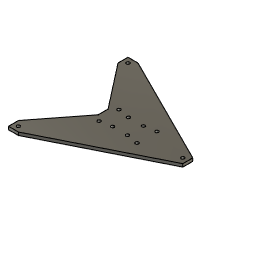
V0.1 Y Carriage (Autodesk Fusion 360 design; units mm, degrees)
Autodesk Fusion 360 part; units mm, degrees
sketch "Sketch1" plane through (0, 0, 0) normal (0, 0, 1) x (1, 0, 0)
  line L0 (60, -60) -> (-60, -60)
  line L1 (-60, -60) -> (-60, 60)
  line L2 (-60, 60) -> (60, 60)
  line L3 (60, 60) -> (60, -60)
  line L4 (60, -60) -> (-60, 60) construction
  line L5 (-60, -60) -> (60, 60) construction
  line L6 (25, 20) -> (-25, 20)
  line L7 (-25, 20) -> (-25, -20)
  line L8 (-25, -20) -> (25, -20)
  line L9 (25, -20) -> (25, 20)
  line L10 (25, 20) -> (-25, -20) construction
  line L11 (-25, 20) -> (25, -20) construction
  line L12 (60, 5) -> (-50, 60)
  line L13 (60, -5) -> (-50, -60)
  line L14 (-60, 50) -> (-25, 5)
  line L15 (-60, -50) -> (-25, -5)
  dimension "d1" = 120
  dimension "d2" = 120
  dimension "d6" = 50
  dimension "d7" = 40
  dimension "d29" = 5
  dimension "d30" = 5
  dimension "d31" = 10
  dimension "d34" = 10
  dimension "d41" = 10
  dimension "d42" = 10
  constraint horizontal L0
  constraint perpendicular L0 L1
  constraint parallel L0 L2
  constraint parallel L1 L3
  constraint coincident L4 origin
  constraint coincident L5 origin
  constraint horizontal L6
  constraint perpendicular L6 L7
  constraint parallel L6 L8
  constraint parallel L7 L9
  constraint coincident L10 origin
  constraint coincident L11 origin
  constraint coincident L3 L12.start
  constraint coincident L2 L12.end
  constraint coincident L3 L13.start
  constraint coincident L0 L13.end
  constraint coincident L1 L14.start
  constraint coincident L7 L14.end
  constraint coincident L1 L15.start
  constraint coincident L7 L15.end
  constraint horizontal L13.start L15.end
  constraint horizontal L12.start L14.end
  measures "d1" distance of L1.end L2.end
  measures "d2" distance of L0.end L1.end
  measures "d6" distance of L7.end L8.end
  measures "d7" distance of L6.end L7.end
  measures "d29" vertical distance of origin L12.start
  measures "d30" vertical distance of origin L13.start
  measures "d31" distance of L1.end L12.end
  measures "d34" distance of L0.end L13.end
  measures "d41" distance of L1.end L14.start
  measures "d42" distance of L0.end L15.start
extrude "Extrude1" add sketch "Sketch1" along normal blind 3 contours L0 L1 L2 L3 L6 L7 L8 L9 L12 L13 L14 L15 | L6 L7 L8 L9
sketch "Sketch2" plane through (0, 0, 3) normal (0, 0, 1) x (-1, 0, 0)
  line L0 (60, 50) -> (60, 60)
  line L1 (60, 60) -> (50, 60)
  line L2 (50, 60) -> (-60, 5)
  line L3 (-60, 5) -> (-60, -5)
  line L4 (-60, -5) -> (50, -60)
  line L5 (50, -60) -> (60, -60)
  line L6 (60, -60) -> (60, -50)
  line L7 (25, 5) -> (60, 50)
  line L8 (60, -50) -> (25, -5)
  line L9 (25, -5) -> (25, 5)
  point P0 (-7.5, -8)
  point P1 (19, -10)
  point P2 (7.5, -8)
  point P3 (-7.5, 8)
  point P4 (7.5, 8)
  point P5 (-19, -10)
  point P6 (19, 10)
  point P7 (-19, 10)
  point P8 (55, -55)
  point P9 (-55, 0)
  point P10 (55, 55)
  dimension "d12" = 7.5
  dimension "d13" = 8
  dimension "d14" = 19
  dimension "d15" = 10
  dimension "d18" = 15
  dimension "d19" = 16
  dimension "d22" = -38
  dimension "d23" = 20
  dimension "d47" = 5
  dimension "d48" = 5
  dimension "d49" = 5
  dimension "d50" = 5
  dimension "d51" = 5
  measures "d12" horizontal distance of origin P0
  measures "d13" vertical distance of origin P0
  measures "d14" horizontal distance of origin P1
  measures "d15" vertical distance of origin P1
  measures "d47" horizontal distance of L0.end P10
  measures "d48" vertical distance of L0.end P10
  measures "d49" horizontal distance of L5.end P8
  measures "d50" vertical distance of L5.end P8
  measures "d51" distance of L3 P9
hole "Hole1" at (-19, 10, 3) at (-7.5, 8, 3) at (7.5, 8, 3) at (19, 10, 3) at (19, -10, 3) at (7.5, -8, 3) at (-7.5, -8, 3) at (-19, -10, 3) at (-55, -55, 3) at (55, 0, 3) at (-55, 55, 3) direction (0, 0, -1) diameter 3.2 depth 30 tip angle 118
named bodies: "3_point_y_carriage"
